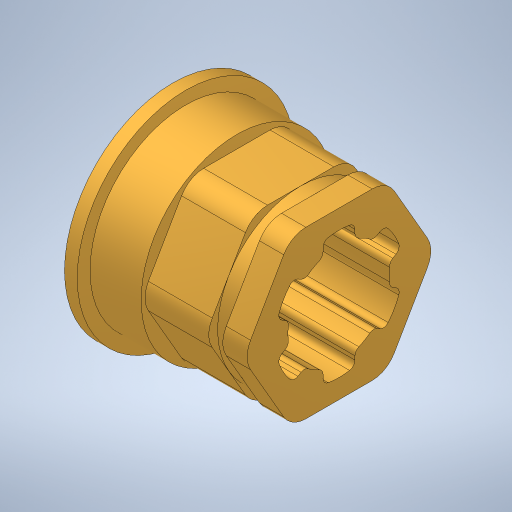
# Autodesk Inventor part: Bushing
Saved by Autodesk Inventor 2023.2 (Build 272271000, 271)
## iProperties
Created: 2024-01-10
Part Number: Bushing
Material: Brass, Soft Yellow
Document SubType Name: Modeling
Designer: Nathan Cai
Mass: 15.747 g
Surface Area: 19.291 cm^2
Volume: 1.85915 cm^3
Density: 8.47 g/cm^3
Appearance: Brass - Satin
Author: Nathan Cai
Autodesk Inventor part; units mm, degrees
ref_plane "YZ Plane" through (0, 0, 0) normal (1, 0, 0) x (0, 1, 0)
ref_plane "XZ Plane" through (0, 0, 0) normal (0, 1, 0) x (-1, 0, 0)
ref_plane "XY Plane" through (0, 0, 0) normal (0, 0, 1) x (1, 0, 0)
sketch "Sketch1" plane through (0, 0, 0) normal (1, 0, 0) x (0, 1, 0)
  circle A0 centre (0, 0) radius 4
  line L0 (4, 0) -> (0, 0) construction
  circle A1 centre (0, 0) radius 6.5 construction
  line L1 (6.5, -3.7528) -> (0, -7.5056)
  line L2 (0, -7.5056) -> (-6.5, -3.7528)
  line L3 (-6.5, -3.7528) -> (-6.5, 3.7528)
  line L4 (-6.5, 3.7528) -> (0, 7.5056)
  line L5 (0, 7.5056) -> (6.5, 3.7528)
  line L6 (6.5, 3.7528) -> (6.5, -3.7528)
  circle A2 centre (0, 0) radius 5
  line L7 (0, 1.25) -> (4.8412, 1.25)
  line L8 (4.8412, 1.25) -> (4.8412, -1.25) construction
  line L9 (4.8412, -1.25) -> (0, -1.25)
  line L10 (0, -1.25) -> (0, 1.25) construction
  line L11 (0, 1.25) -> (4.8412, -1.25) construction
  line L12 (4.8412, 1.25) -> (0, -1.25) construction
  line L13 (-1.0825, 0.625) -> (1.3381, 4.8176)
  line L14 (3.5031, 3.5676) -> (1.0825, -0.625)
  line L15 (-1.0825, -0.625) -> (-3.5031, 3.5676)
  line L16 (-1.3381, 4.8176) -> (1.0825, 0.625)
  line L17 (0, -1.25) -> (-4.8412, -1.25)
  line L18 (-4.8412, 1.25) -> (0, 1.25)
  line L19 (1.0825, -0.625) -> (-1.3381, -4.8176)
  line L20 (-3.5031, -3.5676) -> (-1.0825, 0.625)
  line L21 (1.0825, 0.625) -> (3.5031, -3.5676)
  line L22 (1.3381, -4.8176) -> (-1.0825, -0.625)
  point P0 (6.5, 0)
  point P1 (2.4206, 0)
  point P2 (-3.5031, -3.5676)
  point P3 (-2.9824, -2.6656)
  point P4 (-3.7997, -1.25)
  point P5 (-4.8412, -1.25)
  point P6 (-3.7997, 1.25)
  point P7 (-2.9824, 2.6656)
  point P8 (-1.3381, 4.8176)
  point P9 (-0.8173, 3.9156)
  point P10 (0.8173, 3.9156)
  point P11 (1.3381, 4.8176)
  point P12 (3.5031, 3.5676)
  point P13 (2.9824, 2.6656)
  point P14 (3.7997, 1.25)
  point P15 (4.8412, 1.25)
  point P16 (3.7997, -1.25)
  point P17 (2.9824, -2.6656)
  point P18 (3.5031, -3.5676)
  point P19 (1.3381, -4.8176)
  point P20 (0.8173, -3.9156)
  point P21 (-0.8173, -3.9156)
  point P22 (-1.3381, -4.8176)
  dimension "d0" = 8
  dimension "d28" = 10
  dimension "d5" = 13
  dimension "d29" = 2.5
  dimension "d32" = 360
  constraints: 46 end point, 4 coincident, 4 midpoint, 2 parallel, 2 perpendicular, 2 point on line, 1 centre point, 1 horizontal, 1 tangent, 56 other
  measures "d5" diameter of A1
  measures "d29" distance between parallel lines of L7 L9
extrude "Extrusion1" add sketch "Sketch1" along normal blind 13 contours A0 L14 A2 L7 | L9 A2 L21 A0 | A0 L16 A2 L13 | L22 A2 L19 A0 | A0 L18 A2 L15 | L20 A2 L17 A0 | L1 L2 L3 L4 L5 L6
sketch "Sketch2" plane through (0, 0, 0) normal (-1, 0, 0) x (0, 0, 1)
  circle A0 centre (0, 0) radius 7.5
  line L0 (3.7528, 6.5) -> (7.5056, 0) projected
  line L1 (-3.7528, 6.5) -> (3.7528, 6.5) projected
  line L2 (-7.5056, 0) -> (-3.7528, 6.5) projected
  line L3 (-3.7528, -6.5) -> (-7.5056, 0) projected
  line L4 (3.7528, -6.5) -> (-3.7528, -6.5) projected
  line L5 (7.5056, 0) -> (3.7528, -6.5) projected
  circle A1 centre (0, 0) radius 6.5 construction
  line L6 (-3.7528, -6.5) -> (-7.5056, 0) projected
  line L7 (7.5056, 0) -> (3.7528, -6.5) projected
  line L8 (3.7528, 6.5) -> (7.5056, 0) projected
  line L9 (-3.7528, 6.5) -> (3.7528, 6.5) projected
  line L10 (-7.5056, 0) -> (-3.7528, 6.5) projected
  line L11 (-3.7528, -6.5) -> (-7.5056, 0) projected
  line L12 (3.7528, -6.5) -> (-3.7528, -6.5) projected
  line L13 (7.5056, 0) -> (3.7528, -6.5) projected
  line L14 (-3.5676, -3.5031) -> (-2.6656, -2.9824) projected
  arc A2 (-4.8176, -1.3381) -> (-3.5676, -3.5031) centre (0, 0) ccw projected
  line L15 (-3.9156, -0.8173) -> (-4.8176, -1.3381) projected
  arc A3 (-3.9156, 0.8173) -> (-3.9156, -0.8173) centre (0, 0) ccw projected
  line L16 (-4.8176, 1.3381) -> (-3.9156, 0.8173) projected
  arc A4 (-3.5676, 3.5031) -> (-4.8176, 1.3381) centre (0, 0) ccw projected
  line L17 (-2.6656, 2.9824) -> (-3.5676, 3.5031) projected
  arc A5 (-1.25, 3.7997) -> (-2.6656, 2.9824) centre (0, 0) ccw projected
  line L18 (-1.25, 4.8412) -> (-1.25, 3.7997) projected
  arc A6 (1.25, 4.8412) -> (-1.25, 4.8412) centre (0, 0) ccw projected
  line L19 (1.25, 3.7997) -> (1.25, 4.8412) projected
  arc A7 (2.6656, 2.9824) -> (1.25, 3.7997) centre (0, 0) ccw projected
  line L20 (3.5676, 3.5031) -> (2.6656, 2.9824) projected
  arc A8 (4.8176, 1.3381) -> (3.5676, 3.5031) centre (0, 0) ccw projected
  line L21 (3.9156, 0.8173) -> (4.8176, 1.3381) projected
  arc A9 (3.9156, -0.8173) -> (3.9156, 0.8173) centre (0, 0) ccw projected
  line L22 (4.8176, -1.3381) -> (3.9156, -0.8173) projected
  arc A10 (3.5676, -3.5031) -> (4.8176, -1.3381) centre (0, 0) ccw projected
  line L23 (2.6656, -2.9824) -> (3.5676, -3.5031) projected
  arc A11 (1.25, -3.7997) -> (2.6656, -2.9824) centre (0, 0) ccw projected
  line L24 (1.25, -4.8412) -> (1.25, -3.7997) projected
  arc A12 (-1.25, -4.8412) -> (1.25, -4.8412) centre (0, 0) ccw projected
  line L25 (-1.25, -3.7997) -> (-1.25, -4.8412) projected
  arc A13 (-2.6656, -2.9824) -> (-1.25, -3.7997) centre (0, 0) ccw projected
  dimension "d35" = 15
  constraints: 2 centre point, 2 coincident, 2 tangent
  measures "d35" diameter of A0
extrude "Extrusion2" add sketch "Sketch2" against normal blind 5 contours A0 L5 L4 L3 L2 L1 L0 | L0 A0 | A0 L5 | L1 A0 | A0 L4 | L2 A0 | A0 L3
fillet "Fillet2" radius 0.5 24 edges at (6.5, 4.8412, -1.25) (6.5, 3.7997, -1.25) (6.5, 2.9824, -2.6656) (6.5, 3.5031, -3.5676) (6.5, 0.8173, -3.9156) (6.5, 1.3381, -4.8176) (6.5, -0.8173, -3.9156) (6.5, -1.3381, -4.8176) (6.5, -3.5031, -3.5676) (6.5, -2.9824, -2.6656) (6.5, -3.7997, -1.25) (6.5, -4.8412, -1.25) (6.5, -4.8412, 1.25) (6.5, -3.7997, 1.25) (6.5, -2.9824, 2.6656) (6.5, -3.5031, 3.5676) (6.5, -1.3381, 4.8176) (6.5, -0.8173, 3.9156) (6.5, 1.3381, 4.8176) (6.5, 0.8173, 3.9156) (6.5, 3.5031, 3.5676) (6.5, 2.9824, 2.6656) (6.5, 3.7997, 1.25) (6.5, 4.8412, 1.25)
fillet "Fillet1" radius 2 6 edges at (6.5, 6.5, 3.7528) (6.5, 6.5, -3.7528) (6.5, 0, 7.5056) (6.5, -6.5, 3.7528) (6.5, -6.5, -3.7528) (6.5, 0, -7.5056)
ref_plane "Work Plane1" through (7, 0, 0) normal (1, 0, 0) x (0, 0, -1)
sketch "Sketch4" plane through (0, 0, 0) normal (-1, 0, 0) x (0, 0, 1)
  circle A0 centre (0, 0) radius 7.5 projected
  circle A1 centre (0, 0) radius 8.5
  point P0 (0, 0)
  dimension "d20" = 1
  constraints: 1 centre point
  measures "d20" radial gap between concentric circles of A0 A1
extrude "Extrusion4" add sketch "Sketch4" against normal blind 1
ref_plane "Work Plane2" through (10, 0, 0) normal (1, 0, 0) x (0, 0, -1)
sketch "Sketch5" plane through (10, 0, 0) normal (1, 0, 0) x (0, 0, -1)
  circle A0 centre (0, 0) radius 6.5
  circle A1 centre (0, 0) radius 12.5
  dimension "d24" = 13
  dimension "d25" = 25
  constraints: 2 centre point, 2 coincident
  measures "d24" diameter of A0
  measures "d25" diameter of A1
extrude "Extrusion5" cut sketch "Sketch5" along normal blind 1.1
body "Solid1"
